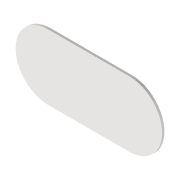
# Autodesk Inventor part: Bauteil3
Saved by Autodesk Inventor 2021 (Build 250183000, 183)
## iProperties
Created: 2021-09-11
Part Number: Bauteil3
Material: Generisch
Document SubType Name: Modeling
Designer: Rama
Density: 1 g/cm^3
Appearance: Vorgabe
Author: Rama
Autodesk Inventor part; units mm, degrees
ref_plane "YZ Plane" through (0, 0, 0) normal (1, 0, 0) x (0, 1, 0)
ref_plane "XZ Plane" through (0, 0, 0) normal (0, 1, 0) x (-1, 0, 0)
sketch "Skizze1" plane through (0, 0, 0) normal (0, 0, 1) x (1, 0, 0)
  circle A0 centre (-91.2697, 43.964) radius 25
  circle A1 centre (-29.2697, 43.964) radius 25
  ellipse E0 centre (-9.1617, 66.4648) end of major axis (16.2819, 71.5914) minor radius 22.416 (-7.6926, 89.0293) -> (-19.3363, 86.6652) ccw projected
  ellipse E1 centre (-31.2859, 110.7263) end of major axis (-1.1112, 117.4506) minor radius 26.6674 (-31.9836, 83.8645) -> (-19.3363, 86.6652) ccw projected
  line L0 (-34.4882, 83.8645) -> (-31.9836, 83.8645) projected
  ellipse E2 centre (-35.1859, 110.7263) end of major axis (-5.0113, 104.0019) minor radius 26.6674 (-47.1355, 86.6652) -> (-34.4882, 83.8645) ccw projected
  ellipse E3 centre (-57.311, 66.4601) end of major axis (-31.8648, 61.3331) minor radius 22.4208 (-47.1355, 86.6652) -> (-58.7792, 89.0293) ccw projected
  line L1 (-61.3973, 89.0293) -> (-58.7792, 89.0293) projected
  ellipse E4 centre (-62.8661, 66.4649) end of major axis (-37.4224, 71.5906) minor radius 22.416 (-61.3973, 89.0293) -> (-73.0392, 86.6659) ccw projected
  ellipse E5 centre (-84.9938, 110.7412) end of major axis (-54.802, 117.4681) minor radius 26.6822 (-85.6923, 83.8645) -> (-73.0392, 86.6659) ccw projected
  line L2 (-88.1968, 83.8645) -> (-85.6923, 83.8645) projected
  ellipse E6 centre (-88.8953, 110.7412) end of major axis (-58.7036, 104.0144) minor radius 26.6822 (-100.8499, 86.6659) -> (-88.1968, 83.8645) ccw projected
  ellipse E7 centre (-111.0239, 66.4602) end of major axis (-85.5776, 61.3339) minor radius 22.4208 (-100.8499, 86.6659) -> (-112.4918, 89.0293) ccw projected
  line L3 (-120.1896, 89.0293) -> (-112.4918, 89.0293) projected
  line L4 (-120.1896, 25.9867) -> (-120.1896, 89.0293) projected
  line L5 (-105.8047, 1.087) -> (-120.1896, 25.9867) projected
  spline S0 degree 3 poles (-103.9219, 0) (-104.0107, 0) (-104.0979, 0.0044) (-104.1833, 0.0134) (-104.269, 0.0223) (-104.353, 0.0358) (-104.4349, 0.0538) (-104.517, 0.0718) (-104.597, 0.0944) (-104.6748, 0.1214) (-104.7529, 0.1485) (-104.8286, 0.1801) (-104.9018, 0.2161) (-104.941, 0.2354) (-104.9795, 0.2559) (-105.0172, 0.2777) (-105.0875, 0.3183) (-105.1555, 0.3634) (-105.2209, 0.4129) (-105.2859, 0.4621) (-105.3484, 0.5156) (-105.408, 0.5733) (-105.4675, 0.6308) (-105.5243, 0.6924) (-105.5781, 0.758) (-105.6317, 0.8233) (-105.6824, 0.8925) (-105.7301, 0.9654) (-105.7558, 1.0049) (-105.7807, 1.0454) (-105.8047, 1.087) knots -2.338618 -2.338618 -2.338618 -2.338618 -2.082467 -2.082467 -2.082467 -1.825195 -1.825195 -1.825195 -1.567203 -1.567203 -1.567203 -1.307968 -1.307968 -1.307968 -1.168939 -1.168939 -1.168939 -0.909645 -0.909645 -0.909645 -0.651775 -0.651775 -0.651775 -0.394667 -0.394667 -0.394667 -0.138517 -0.138517 -0.138517 0 0 0 0 projected
  line L6 (-16.2642, 0) -> (-103.9219, 0) projected
  spline S1 degree 3 poles (-14.3814, 1.087) (-14.4258, 1.0102) (-14.4732, 0.9369) (-14.5236, 0.8675) (-14.5742, 0.7977) (-14.6278, 0.7318) (-14.6843, 0.6699) (-14.7409, 0.6078) (-14.8004, 0.5498) (-14.8626, 0.496) (-14.9251, 0.442) (-14.9903, 0.3922) (-15.058, 0.3468) (-15.0943, 0.3225) (-15.1313, 0.2995) (-15.169, 0.2777) (-15.2393, 0.2371) (-15.3124, 0.2007) (-15.388, 0.1688) (-15.4632, 0.137) (-15.5408, 0.1097) (-15.6206, 0.0868) (-15.7002, 0.064) (-15.782, 0.0457) (-15.8657, 0.0318) (-15.9491, 0.018) (-16.0345, 0.0087) (-16.1216, 0.0039) (-16.1686, 0.0013) (-16.2162, 0) (-16.2642, 0) knots -2.338618 -2.338618 -2.338618 -2.338618 -2.08263 -2.08263 -2.08263 -1.82552 -1.82552 -1.82552 -1.567689 -1.567689 -1.567689 -1.308614 -1.308614 -1.308614 -1.169679 -1.169679 -1.169679 -0.910226 -0.910226 -0.910226 -0.652194 -0.652194 -0.652194 -0.394923 -0.394923 -0.394923 -0.138612 -0.138612 -0.138612 0 0 0 0 projected
  line L7 (0.0001, 26.012) -> (-14.3814, 1.087) projected
  line L8 (0, 89.0293) -> (0.0001, 26.012) projected
  line L9 (-7.6926, 89.0293) -> (0, 89.0293) projected
  circle A2 centre (-64.1021, 9.6247) radius 1.6 projected
  circle A3 centre (-56.1021, 9.6247) radius 1.6 projected
  arc A4 (-20.5619, 52.6116) -> (-33.7385, 60.9564) centre (-35.5323, 43.5486) ccw projected
  arc A5 (-20.5619, 52.6116) -> (-29.2715, 52.6538) centre (-24.9939, 36.718) ccw projected
  arc A6 (-29.2715, 52.6538) -> (-38.5147, 54.1885) centre (-35.5323, 43.5486) ccw projected
  arc A7 (-33.7385, 60.9564) -> (-38.5147, 54.1885) centre (-24.3476, 49.2598) ccw projected
  arc A8 (-40.2873, 53.5232) -> (-46.2379, 46.2856) centre (-35.5323, 43.5486) ccw projected
  arc A9 (-49.711, 53.806) -> (-46.2379, 46.2856) centre (-34.8859, 56.0904) ccw projected
  arc A10 (-35.8959, 61.0448) -> (-49.711, 53.806) centre (-35.5323, 43.5486) ccw projected
  arc A11 (-35.8959, 61.0448) -> (-40.2873, 53.5232) centre (-24.3476, 49.2598) ccw projected
  arc A12 (-50.8662, 51.9818) -> (-51.5048, 36.3981) centre (-35.5323, 43.5486) ccw projected
  arc A13 (-50.8662, 51.9818) -> (-46.548, 44.4179) centre (-34.8859, 56.0904) ccw projected
  arc A14 (-46.548, 44.4179) -> (-43.2554, 35.6457) centre (-35.5323, 43.5486) ccw projected
  arc A15 (-51.5048, 36.3981) -> (-43.2554, 35.6457) centre (-46.0706, 50.3792) ccw projected
  arc A16 (-50.5026, 34.4856) -> (-37.326, 26.1408) centre (-35.5323, 43.5486) ccw projected
  arc A17 (-50.5026, 34.4856) -> (-41.793, 34.4433) centre (-46.0706, 50.3792) ccw projected
  arc A18 (-41.793, 34.4433) -> (-32.5498, 32.9087) centre (-35.5323, 43.5486) ccw projected
  arc A19 (-37.326, 26.1408) -> (-32.5498, 32.9087) centre (-46.7169, 37.8374) ccw projected
  arc A20 (-30.7773, 33.574) -> (-24.8266, 40.8115) centre (-35.5323, 43.5486) ccw projected
  arc A21 (-21.3535, 33.2912) -> (-24.8266, 40.8115) centre (-36.1786, 31.0068) ccw projected
  arc A22 (-35.1686, 26.0524) -> (-21.3535, 33.2912) centre (-35.5323, 43.5486) ccw projected
  arc A23 (-35.1686, 26.0524) -> (-30.7773, 33.574) centre (-46.7169, 37.8374) ccw projected
  arc A24 (-24.5165, 42.6792) -> (-27.8091, 51.4514) centre (-35.5323, 43.5486) ccw projected
  arc A25 (-19.5597, 50.699) -> (-27.8091, 51.4514) centre (-24.9939, 36.718) ccw projected
  arc A26 (-20.1983, 35.1154) -> (-19.5597, 50.699) centre (-35.5323, 43.5486) ccw projected
  arc A27 (-20.1983, 35.1154) -> (-24.5165, 42.6792) centre (-36.1786, 31.0068) ccw projected
  arc A28 (-87.0592, 33.5737) -> (-81.1083, 40.811) centre (-91.8139, 43.5484) ccw projected
  arc A29 (-77.6355, 33.2906) -> (-81.1083, 40.811) centre (-92.4606, 31.0066) ccw projected
  arc A30 (-91.4508, 26.0522) -> (-77.6355, 33.2906) centre (-91.8139, 43.5484) ccw projected
  arc A31 (-91.4508, 26.0522) -> (-87.0592, 33.5737) centre (-102.9987, 37.8376) ccw projected
  arc A32 (-106.7845, 34.4859) -> (-93.6082, 26.1406) centre (-91.8139, 43.5484) ccw projected
  arc A33 (-106.7845, 34.4859) -> (-98.0749, 34.4434) centre (-102.352, 50.3794) ccw projected
  arc A34 (-98.0749, 34.4434) -> (-88.8318, 32.9084) centre (-91.8139, 43.5484) ccw projected
  arc A35 (-93.6082, 26.1406) -> (-88.8318, 32.9084) centre (-102.9987, 37.8376) ccw projected
  arc A36 (-76.8432, 52.6109) -> (-90.0195, 60.9562) centre (-91.8139, 43.5484) ccw projected
  arc A37 (-76.8432, 52.6109) -> (-85.5528, 52.6534) centre (-81.2757, 36.7174) ccw projected
  arc A38 (-85.5528, 52.6534) -> (-94.796, 54.1884) centre (-91.8139, 43.5484) ccw projected
  arc A39 (-90.0195, 60.9562) -> (-94.796, 54.1884) centre (-80.629, 49.2592) ccw projected
  arc A40 (-96.5686, 53.5231) -> (-102.5194, 46.2858) centre (-91.8139, 43.5484) ccw projected
  arc A41 (-105.9923, 53.8062) -> (-102.5194, 46.2858) centre (-91.1672, 56.0902) ccw projected
  arc A42 (-92.1769, 61.0446) -> (-105.9923, 53.8062) centre (-91.8139, 43.5484) ccw projected
  arc A43 (-92.1769, 61.0446) -> (-96.5686, 53.5231) centre (-80.629, 49.2592) ccw projected
  arc A44 (-80.7982, 42.6787) -> (-84.0904, 51.451) centre (-91.8139, 43.5484) ccw projected
  arc A45 (-75.8411, 50.6983) -> (-84.0904, 51.451) centre (-81.2757, 36.7174) ccw projected
  arc A46 (-76.4802, 35.1147) -> (-75.8411, 50.6983) centre (-91.8139, 43.5484) ccw projected
  arc A47 (-76.4802, 35.1147) -> (-80.7982, 42.6787) centre (-92.4606, 31.0066) ccw projected
  arc A48 (-107.1476, 51.9821) -> (-107.7866, 36.3985) centre (-91.8139, 43.5484) ccw projected
  arc A49 (-107.1476, 51.9821) -> (-102.8296, 44.4181) centre (-91.1672, 56.0902) ccw projected
  arc A50 (-102.8296, 44.4181) -> (-99.5373, 35.6458) centre (-91.8139, 43.5484) ccw projected
  arc A51 (-107.7866, 36.3985) -> (-99.5373, 35.6458) centre (-102.352, 50.3794) ccw projected
  arc A52 (-86.0548, 46.6926) -> (-85.9137, 46.6766) centre (-85.9683, 46.825) ccw projected
  line L10 (-85.6942, 46.741) -> (-85.9156, 46.6796) projected
  spline S2 degree 3 poles (-84.7234, 46.8312) (-84.8974, 46.8308) (-85.0866, 46.8262) (-85.2632, 46.8106) (-85.4061, 46.798) (-85.5539, 46.7772) (-85.6942, 46.741) knots -0.122826 -0.122826 -0.122826 -0.122826 -0.054961 -0.054961 -0.054961 0 0 0 0 projected
  spline S3 degree 3 poles (-83.2154, 46.6804) (-83.3883, 46.7327) (-83.5805, 46.7673) (-83.7805, 46.7898) (-83.7975, 46.7917) (-83.8146, 46.7936) (-83.8318, 46.7953) (-83.8434, 46.7965) (-83.855, 46.7976) (-83.8666, 46.7987) (-84.1413, 46.8249) (-84.4269, 46.8312) (-84.6873, 46.8312) (-84.6994, 46.8312) (-84.7114, 46.8312) (-84.7234, 46.8312) knots -0.194136 -0.194136 -0.194136 -0.194136 -0.118483 -0.118483 -0.118483 -0.112036 -0.112036 -0.112036 -0.107675 -0.107675 -0.107675 -0.004775 -0.004775 -0.004775 0 0 0 0 projected
  spline S4 degree 3 poles (-82.3446, 45.9479) (-82.3857, 46.0372) (-82.437, 46.121) (-82.4975, 46.1985) (-82.5463, 46.261) (-82.6007, 46.3188) (-82.6596, 46.3715) (-82.6735, 46.3839) (-82.6877, 46.3961) (-82.7021, 46.4079) (-82.8528, 46.5322) (-83.0284, 46.6239) (-83.2154, 46.6804) knots -1.489588 -1.489588 -1.489588 -1.489588 -1.116559 -1.116559 -1.116559 -0.815384 -0.815384 -0.815384 -0.744362 -0.744362 -0.744362 0 0 0 0 projected
  spline S5 degree 3 poles (-82.1303, 44.589) (-82.1309, 44.8596) (-82.1416, 45.1087) (-82.1774, 45.3502) (-82.1791, 45.3619) (-82.1809, 45.3736) (-82.1827, 45.3853) (-82.214, 45.5816) (-82.2649, 45.7746) (-82.3446, 45.9479) knots -0.151678 -0.151678 -0.151678 -0.151678 -0.0703 -0.0703 -0.0703 -0.066352 -0.066352 -0.066352 0 0 0 0 projected
  line L11 (-82.1256, 42.5169) -> (-82.1303, 44.589) projected
  spline S6 degree 3 poles (-82.7841, 40.9566) (-82.6707, 41.0392) (-82.5715, 41.1365) (-82.4867, 41.2485) (-82.4227, 41.3332) (-82.3687, 41.4239) (-82.3236, 41.5186) (-82.3144, 41.5381) (-82.3055, 41.5577) (-82.297, 41.5774) (-82.2917, 41.5898) (-82.2865, 41.6022) (-82.2814, 41.6147) (-82.1669, 41.8986) (-82.1249, 42.2114) (-82.1256, 42.5169) knots -0.223192 -0.223192 -0.223192 -0.223192 -0.170194 -0.170194 -0.170194 -0.130156 -0.130156 -0.130156 -0.121953 -0.121953 -0.121953 -0.11681 -0.11681 -0.11681 0 0 0 0 projected
  spline S7 degree 3 poles (-84.6323, 40.5153) (-84.1659, 40.5163) (-83.7588, 40.5549) (-83.398, 40.6621) (-83.3923, 40.6638) (-83.3865, 40.6656) (-83.3808, 40.6673) (-83.3748, 40.6691) (-83.3688, 40.671) (-83.3629, 40.6728) (-83.1669, 40.7342) (-82.9646, 40.825) (-82.7841, 40.9566) knots -2.452794 -2.452794 -2.452794 -2.452794 -0.895722 -0.895722 -0.895722 -0.870966 -0.870966 -0.870966 -0.845148 -0.845148 -0.845148 0 0 0 0 projected
  spline S8 degree 3 poles (-85.5377, 40.5812) (-85.4045, 40.5549) (-85.2653, 40.5393) (-85.1305, 40.5298) (-84.9669, 40.5183) (-84.7951, 40.5149) (-84.6323, 40.5153) knots -0.112604 -0.112604 -0.112604 -0.112604 -0.061749 -0.061749 -0.061749 0 0 0 0 projected
  line L12 (-85.7322, 40.6271) -> (-85.5377, 40.5812) projected
  arc A53 (-85.731, 40.6295) -> (-85.9362, 40.4782) centre (-85.7781, 40.4786) ccw projected
  line L13 (-85.9315, 38.412) -> (-85.9362, 40.4782) projected
  arc A54 (-86.0893, 38.2535) -> (-85.9315, 38.412) centre (-86.0896, 38.4116) ccw projected
  line L14 (-88.1643, 38.2488) -> (-86.0893, 38.2535) projected
  arc A55 (-88.3228, 38.4065) -> (-88.1643, 38.2488) centre (-88.1646, 38.4069) ccw projected
  line L15 (-88.3413, 46.5552) -> (-88.3228, 38.4065) projected
  arc A56 (-88.1835, 46.7137) -> (-88.3413, 46.5552) centre (-88.1832, 46.5556) ccw projected
  line L16 (-86.1416, 46.7183) -> (-88.1835, 46.7137) projected
  arc A57 (-86.0548, 46.6926) -> (-86.1416, 46.7183) centre (-86.1413, 46.5602) ccw projected
  line L17 (-92.4601, 40.7652) -> (-92.4716, 44.6753) projected
  arc A58 (-92.6179, 40.6067) -> (-92.4601, 40.7652) centre (-92.6182, 40.7648) ccw projected
  line L18 (-94.6929, 40.602) -> (-92.6179, 40.6067) projected
  arc A59 (-94.8514, 40.7598) -> (-94.6929, 40.602) centre (-94.6932, 40.7601) ccw projected
  line L19 (-94.8645, 46.5404) -> (-94.8514, 40.7598) projected
  arc A60 (-94.7068, 46.6989) -> (-94.8645, 46.5404) centre (-94.7064, 46.5407) ccw projected
  line L20 (-92.6405, 46.7036) -> (-94.7068, 46.6989) projected
  arc A61 (-92.5441, 46.6711) -> (-92.6405, 46.7036) centre (-92.6402, 46.5454) ccw projected
  arc A62 (-92.5441, 46.6711) -> (-92.3949, 46.6478) centre (-92.4481, 46.7967) ccw projected
  spline S9 degree 3 poles (-91.1918, 46.8165) (-91.4073, 46.816) (-91.63, 46.8056) (-92.0309, 46.7513) (-92.2173, 46.7112) (-92.3949, 46.6478) knots -0.153916 -0.153916 -0.153916 -0.153916 -0.071551 -0.071551 0 0 0 0 projected
  spline S10 degree 3 poles (-89.4966, 46.3526) (-89.5966, 46.4414) (-89.7069, 46.5144) (-89.8263, 46.5738) (-89.9507, 46.6358) (-90.0821, 46.6814) (-90.2086, 46.7143) (-90.2124, 46.7153) (-90.2162, 46.7162) (-90.22, 46.7172) (-90.5157, 46.7925) (-90.8412, 46.8173) (-91.1918, 46.8165) knots -0.256586 -0.256586 -0.256586 -0.256586 -0.19968 -0.19968 -0.19968 -0.140397 -0.140397 -0.140397 -0.138614 -0.138614 -0.138614 0 0 0 0 projected
  spline S11 degree 3 poles (-88.9503, 44.9024) (-88.9507, 45.0851) (-88.9666, 45.2696) (-89.004, 45.4486) (-89.0386, 45.6139) (-89.0919, 45.7756) (-89.1694, 45.9264) (-89.2524, 46.0878) (-89.3607, 46.2317) (-89.4966, 46.3526) knots -0.202492 -0.202492 -0.202492 -0.202492 -0.132951 -0.132951 -0.132951 -0.068717 -0.068717 -0.068717 0 0 0 0 projected
  line L21 (-88.9409, 40.7732) -> (-88.9503, 44.9024) projected
  arc A63 (-89.0986, 40.6147) -> (-88.9409, 40.7732) centre (-89.099, 40.7729) ccw projected
  line L22 (-91.1736, 40.61) -> (-89.0986, 40.6147) projected
  arc A64 (-91.3321, 40.7678) -> (-91.1736, 40.61) centre (-91.174, 40.7681) ccw projected
  line L23 (-91.3387, 44.6778) -> (-91.3321, 40.7678) projected
  line L24 (-91.3482, 44.8676) -> (-91.3387, 44.6778) projected
  arc A65 (-91.3508, 44.8669) -> (-91.4873, 45.0072) centre (-91.508, 44.8504) ccw projected
  line L25 (-91.8017, 45.0269) -> (-91.4852, 45.0129) projected
  spline S12 degree 3 poles (-92.3289, 44.9918) (-92.2912, 44.9983) (-92.2427, 45.0046) (-92.1896, 45.0097) (-92.1778, 45.0108) (-92.1658, 45.0119) (-92.1537, 45.0129) (-92.1468, 45.0135) (-92.1398, 45.014) (-92.1327, 45.0146) (-92.1287, 45.0149) (-92.1247, 45.0152) (-92.1207, 45.0155) (-92.0101, 45.0237) (-91.904, 45.0266) (-91.8017, 45.0269) knots -0.073532 -0.073532 -0.073532 -0.073532 -0.052029 -0.052029 -0.052029 -0.047253 -0.047253 -0.047253 -0.044506 -0.044506 -0.044506 -0.042944 -0.042944 -0.042944 0 0 0 0 projected
  arc A66 (-92.3289, 44.9918) -> (-92.4591, 44.8544) centre (-92.302, 44.8359) ccw projected
  line L26 (-92.4716, 44.6753) -> (-92.4619, 44.8553) projected
  spline S13 degree 3 poles (-100.0607, 46.5983) (-100.1975, 46.5563) (-100.333, 46.5049) (-100.4611, 46.4399) (-100.5808, 46.3793) (-100.6936, 46.3071) (-100.7961, 46.22) knots -0.105465 -0.105465 -0.105465 -0.105465 -0.050938 -0.050938 -0.050938 0 0 0 0 projected
  ellipse E8 centre (-104.9794, 13.7975) end of major axis (-111.7131, -19.1173) minor radius 10.4703 (-99.2435, 46.7635) -> (-100.0607, 46.5983) ccw projected
  spline S14 degree 3 poles (-98.4166, 46.8001) (-98.5634, 46.7997) (-98.7129, 46.797) (-98.8596, 46.7906) (-98.9869, 46.785) (-99.1167, 46.7764) (-99.2435, 46.7635) knots -0.104179 -0.104179 -0.104179 -0.104179 -0.048423 -0.048423 -0.048423 0 0 0 0 projected
  spline S15 degree 3 poles (-97.5646, 46.767) (-97.6917, 46.7799) (-97.8237, 46.7878) (-97.9513, 46.7927) (-98.1047, 46.7985) (-98.2633, 46.8004) (-98.4166, 46.8001) knots -0.106414 -0.106414 -0.106414 -0.106414 -0.058092 -0.058092 -0.058092 0 0 0 0 projected
  spline S16 degree 3 poles (-96.8203, 46.6251) (-96.8656, 46.6373) (-96.9895, 46.67) (-97.1252, 46.6983) (-97.1375, 46.7008) (-97.1498, 46.7033) (-97.1622, 46.7058) (-97.175, 46.7084) (-97.1879, 46.7109) (-97.2007, 46.7133) (-97.3361, 46.7392) (-97.4502, 46.7554) (-97.5646, 46.767) knots -0.117674 -0.117674 -0.117674 -0.117674 -0.063481 -0.063481 -0.063481 -0.05859 -0.05859 -0.05859 -0.053521 -0.053521 -0.053521 0 0 0 0 projected
  spline S17 degree 3 poles (-96.034, 46.2358) (-96.1264, 46.3132) (-96.2261, 46.3802) (-96.3483, 46.4438) (-96.3632, 46.4515) (-96.3785, 46.4592) (-96.3941, 46.4669) (-96.4026, 46.471) (-96.4111, 46.4751) (-96.4197, 46.4791) (-96.5834, 46.5564) (-96.7598, 46.6084) (-96.8203, 46.6251) knots -0.039747 -0.039747 -0.039747 -0.039747 -0.023556 -0.023556 -0.023556 -0.021582 -0.021582 -0.021582 -0.020509 -0.020509 -0.020509 0 0 0 0 projected
  spline S18 degree 3 poles (-95.5204, 45.5204) (-95.5821, 45.6592) (-95.6555, 45.7936) (-95.7435, 45.9178) (-95.827, 46.0355) (-95.9231, 46.143) (-96.034, 46.2358) knots -0.112543 -0.112543 -0.112543 -0.112543 -0.05478 -0.05478 -0.05478 0 0 0 0 projected
  spline S19 degree 3 poles (-95.3191, 44.4823) (-95.3195, 44.6658) (-95.3337, 44.8506) (-95.368, 45.0313) (-95.3999, 45.1998) (-95.4491, 45.3641) (-95.5204, 45.5204) knots -0.134887 -0.134887 -0.134887 -0.134887 -0.065077 -0.065077 -0.065077 0 0 0 0 projected
  line L27 (-95.3155, 42.9145) -> (-95.3191, 44.4823) projected
  spline S20 degree 3 poles (-95.5079, 41.8411) (-95.4399, 42.0053) (-95.3924, 42.1764) (-95.3615, 42.3512) (-95.3288, 42.537) (-95.3151, 42.7261) (-95.3155, 42.9145) knots -0.13893 -0.13893 -0.13893 -0.13893 -0.071582 -0.071582 -0.071582 0 0 0 0 projected
  spline S21 degree 3 poles (-96.0477, 41.0725) (-95.9525, 41.1522) (-95.8705, 41.2309) (-95.7725, 41.3655) (-95.7668, 41.3732) (-95.7611, 41.3811) (-95.7554, 41.3892) (-95.7497, 41.3972) (-95.744, 41.4054) (-95.7382, 41.4137) (-95.6344, 41.5631) (-95.5661, 41.7005) (-95.5079, 41.8411) knots -1.203844 -1.203844 -1.203844 -1.203844 -0.643218 -0.643218 -0.643218 -0.61089 -0.61089 -0.61089 -0.578662 -0.578662 -0.578662 0 0 0 0 projected
  spline S22 degree 3 poles (-96.7812, 40.6888) (-96.6732, 40.7251) (-96.5657, 40.7659) (-96.4452, 40.8239) (-96.4247, 40.8337) (-96.4039, 40.844) (-96.3827, 40.855) (-96.3741, 40.8595) (-96.3655, 40.864) (-96.357, 40.8685) (-96.3288, 40.8836) (-96.3013, 40.899) (-96.2751, 40.9145) (-96.255, 40.9264) (-96.2358, 40.9382) (-96.2175, 40.9499) (-96.1355, 41.002) (-96.0756, 41.0498) (-96.0477, 41.0725) knots -0.034306 -0.034306 -0.034306 -0.034306 -0.020192 -0.020192 -0.020192 -0.017794 -0.017794 -0.017794 -0.016819 -0.016819 -0.016819 -0.013578 -0.013578 -0.013578 -0.011102 -0.011102 -0.011102 0 0 0 0 projected
  spline S23 degree 3 poles (-97.6176, 40.5086) (-97.6088, 40.5094) (-97.598, 40.5104) (-97.5853, 40.5117) (-97.5723, 40.513) (-97.5572, 40.5146) (-97.5405, 40.5165) (-97.4857, 40.5227) (-97.4123, 40.5327) (-97.3322, 40.5469) (-97.311, 40.5507) (-97.2894, 40.5547) (-97.2675, 40.559) (-97.2456, 40.5633) (-97.2236, 40.5679) (-97.2014, 40.5727) (-97.0458, 40.6063) (-96.9188, 40.6431) (-96.7943, 40.6844) (-96.79, 40.6859) (-96.7856, 40.6873) (-96.7812, 40.6888) knots -0.135222 -0.135222 -0.135222 -0.135222 -0.125386 -0.125386 -0.125386 -0.115191 -0.115191 -0.115191 -0.081826 -0.081826 -0.081826 -0.073 -0.073 -0.073 -0.064174 -0.064174 -0.064174 -0.002177 -0.002177 -0.002177 0 0 0 0 projected
  line L28 (-98.4023, 40.4839) -> (-97.6176, 40.5086) projected
  spline S24 degree 3 poles (-99.2439, 40.5111) (-99.1214, 40.5002) (-98.992, 40.4938) (-98.8691, 40.4899) (-98.7159, 40.485) (-98.5554, 40.4836) (-98.4023, 40.4839) knots -0.104414 -0.104414 -0.104414 -0.104414 -0.057924 -0.057924 -0.057924 0 0 0 0 projected
  spline S25 degree 3 poles (-99.9858, 40.6616) (-99.8604, 40.6239) (-99.7328, 40.5908) (-99.6045, 40.5646) (-99.4855, 40.5403) (-99.365, 40.5218) (-99.2439, 40.5111) knots -0.095821 -0.095821 -0.095821 -0.095821 -0.046096 -0.046096 -0.046096 0 0 0 0 projected
  spline S26 degree 3 poles (-100.7691, 41.0652) (-100.6711, 40.9828) (-100.5652, 40.9113) (-100.4363, 40.8433) (-100.4276, 40.8387) (-100.4188, 40.8342) (-100.4099, 40.8296) (-100.4012, 40.8252) (-100.3926, 40.8209) (-100.384, 40.8166) (-100.2927, 40.7712) (-100.2105, 40.7367) (-100.1351, 40.7099) (-100.0833, 40.6915) (-100.0345, 40.6763) (-99.9858, 40.6616) knots -1.124833 -1.124833 -1.124833 -1.124833 -0.63928 -0.63928 -0.63928 -0.606632 -0.606632 -0.606632 -0.574712 -0.574712 -0.574712 -0.234192 -0.234192 -0.234192 0 0 0 0 projected
  spline S27 degree 3 poles (-101.3001, 41.7998) (-101.2554, 41.7025) (-101.2064, 41.6013) (-101.1311, 41.4851) (-101.1183, 41.4652) (-101.1047, 41.445) (-101.0905, 41.4245) (-101.083, 41.4136) (-101.0753, 41.4026) (-101.0674, 41.3915) (-100.9728, 41.2592) (-100.8771, 41.156) (-100.7691, 41.0652) knots -0.13558 -0.13558 -0.13558 -0.13558 -0.077687 -0.077687 -0.077687 -0.067813 -0.067813 -0.067813 -0.062578 -0.062578 -0.062578 0 0 0 0 projected
  spline S28 degree 3 poles (-101.5001, 42.9004) (-101.4997, 42.7177) (-101.4895, 42.5333) (-101.451, 42.3181) (-101.4489, 42.3061) (-101.4468, 42.2943) (-101.4446, 42.2828) (-101.4252, 42.1792) (-101.4039, 42.0906) (-101.3802, 42.014) (-101.3564, 41.9369) (-101.33, 41.871) (-101.3001, 41.7998) knots -0.100587 -0.100587 -0.100587 -0.100587 -0.051574 -0.051574 -0.051574 -0.04885 -0.04885 -0.04885 -0.024504 -0.024504 -0.024504 0 0 0 0 projected
  line L29 (-101.5036, 44.4682) -> (-101.5001, 42.9004) projected
  spline S29 degree 3 poles (-101.3161, 45.4901) (-101.321, 45.4778) (-101.3258, 45.4658) (-101.3303, 45.4541) (-101.3347, 45.4429) (-101.3389, 45.432) (-101.343, 45.4212) (-101.3467, 45.4114) (-101.3503, 45.4018) (-101.3538, 45.3923) (-101.387, 45.3019) (-101.4147, 45.2072) (-101.4366, 45.1107) (-101.4447, 45.0752) (-101.452, 45.0394) (-101.4585, 45.0035) (-101.4905, 44.8269) (-101.504, 44.6473) (-101.5036, 44.4682) knots -1.324342 -1.324342 -1.324342 -1.324342 -1.279119 -1.279119 -1.279119 -1.236014 -1.236014 -1.236014 -1.196583 -1.196583 -1.196583 -0.819658 -0.819658 -0.819658 -0.681017 -0.681017 -0.681017 0 0 0 0 projected
  spline S30 degree 3 poles (-100.7961, 46.22) (-100.9097, 46.1253) (-101.0082, 46.0155) (-101.0933, 45.8946) (-101.0987, 45.887) (-101.1039, 45.8794) (-101.1094, 45.8713) (-101.189, 45.7546) (-101.249, 45.6387) (-101.3029, 45.5193) (-101.3073, 45.5096) (-101.3117, 45.4998) (-101.3161, 45.4901) knots -1.146381 -1.146381 -1.146381 -1.146381 -0.585726 -0.585726 -0.585726 -0.550633 -0.550633 -0.550633 -0.041397 -0.041397 -0.041397 0 0 0 0 projected
  line L30 (-34.9505, 49.0872) -> (-34.9505, 47.167) projected
  arc A67 (-34.7875, 49.2502) -> (-34.9505, 49.0872) centre (-34.7875, 49.0872) ccw projected
  line L31 (-32.648, 49.2502) -> (-34.7875, 49.2502) projected
  arc A68 (-32.485, 49.0872) -> (-32.648, 49.2502) centre (-32.648, 49.0872) ccw projected
  line L32 (-32.485, 40.7758) -> (-32.485, 49.0872) projected
  arc A69 (-32.648, 40.6128) -> (-32.485, 40.7758) centre (-32.648, 40.7758) ccw projected
  line L33 (-34.7875, 40.6128) -> (-32.648, 40.6128) projected
  arc A70 (-34.9505, 40.7758) -> (-34.7875, 40.6128) centre (-34.7875, 40.7758) ccw projected
  line L34 (-34.9481, 44.8073) -> (-34.9505, 40.7758) projected
  line L35 (-34.9575, 45.003) -> (-34.9481, 44.8073) projected
  arc A71 (-34.9601, 45.0023) -> (-35.1006, 45.1472) centre (-35.1223, 44.9856) ccw projected
  line L36 (-35.4246, 45.1683) -> (-35.0983, 45.1531) projected
  spline S31 degree 3 poles (-35.9684, 45.1334) (-35.9561, 45.1355) (-35.9427, 45.1375) (-35.9284, 45.1395) (-35.8978, 45.1438) (-35.8629, 45.1478) (-35.826, 45.1513) (-35.8067, 45.1531) (-35.7868, 45.1548) (-35.7668, 45.1563) (-35.7625, 45.1566) (-35.7582, 45.1569) (-35.7539, 45.1573) (-35.6397, 45.1654) (-35.5302, 45.1683) (-35.4246, 45.1683) knots -0.073532 -0.073532 -0.073532 -0.073532 -0.066741 -0.066741 -0.066741 -0.052199 -0.052199 -0.052199 -0.044602 -0.044602 -0.044602 -0.042977 -0.042977 -0.042977 0 0 0 0 projected
  arc A72 (-35.9684, 45.1334) -> (-36.1029, 44.992) centre (-35.9409, 44.9726) ccw projected
  line L37 (-36.1161, 44.8073) -> (-36.1058, 44.9929) projected
  line L38 (-36.1135, 40.7758) -> (-36.1161, 44.8073) projected
  arc A73 (-36.2766, 40.6128) -> (-36.1135, 40.7758) centre (-36.2766, 40.7758) ccw projected
  line L39 (-38.416, 40.6128) -> (-36.2766, 40.6128) projected
  arc A74 (-38.579, 40.7758) -> (-38.416, 40.6128) centre (-38.416, 40.7758) ccw projected
  line L40 (-38.579, 42.6932) -> (-38.579, 40.7758) projected
  arc A75 (-38.579, 42.6932) -> (-38.579, 44.2828) centre (-55.2428, 43.488) ccw projected
  line L41 (-38.579, 46.736) -> (-38.579, 44.2828) projected
  arc A76 (-38.416, 46.899) -> (-38.579, 46.736) centre (-38.416, 46.736) ccw projected
  line L42 (-36.1895, 46.899) -> (-38.416, 46.899) projected
  arc A77 (-36.1062, 46.8761) -> (-36.1895, 46.899) centre (-36.1895, 46.736) ccw projected
  arc A78 (-36.1062, 46.8761) -> (-35.9727, 46.8611) centre (-36.0228, 47.0161) ccw projected
  spline S32 degree 3 poles (-35.1051, 47.0042) (-35.2586, 46.9963) (-35.4139, 46.9818) (-35.5658, 46.9571) (-35.7032, 46.9348) (-35.84, 46.9039) (-35.9727, 46.8611) knots -0.108009 -0.108009 -0.108009 -0.108009 -0.05128 -0.05128 -0.05128 0 0 0 0 projected
  arc A79 (-35.1051, 47.0042) -> (-34.9505, 47.167) centre (-35.1135, 47.167) ccw projected
  line L43 (-102.352, 68.964) -> (-17, 68.964)
  line L44 (-102.352, 18.964) -> (-14.3814, 18.964)
  point P0 (0, 0)
  point P1 (-91.2697, 68.964)
  point P2 (-91.2697, 18.964)
  point P3 (-29.2697, 18.964)
  point P4 (-29.2697, 68.964)
  dimension "d0" = 50
  dimension "d1" = 50
  dimension "d2" = 62
  dimension "d3" = 0
  constraints: 4 end point, 3 tangent, 2 centre point, 1 horizontal, 9 other
  measures "d0" diameter of A0
  measures "d1" diameter of A1
  measures "d2" distance of A1.centre A0.centre
  measures "d3" vertical distance of A1.centre A0.centre
ref_plane "Arbeitsebene1" through (-121.3898, -1.0253, -1.7438) normal (0, 0, -1) x (0, 1, 0)
extrude "Extrusion1" add sketch "Skizze1" against normal up to surface (1.7438 mm away) contours A0 | A0 L43 A1 L44 | A1 | A5 A6 A7 A4 | A8 A9 A10 A11 | A13 A14 A15 A12 | A17 A18 A19 A16 | A20 A21 A22 A23 | A24 A25 A26 A27 | A28 A29 A30 A31 | A33 A34 A35 A32 | A37 A38 A39 A36 | A40 A41 A42 A43 | A44 A45 A46 A47 | A49 A50 A51 A48 | E8 S14 S15 S16 S17 S18 S19 L27 S20 S21 S22 S23 L28 S24 S25 S26 S27 S28 L29 S29 S30 S13
equation "\"d1\" = d0"
